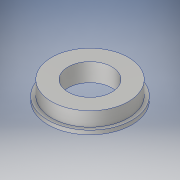
# Autodesk Inventor part: F6801_2019
Saved by Autodesk Inventor 2019.4 (Build 234330000, 330)
## iProperties
Created: 2020-02-07
Part Number: F6801_2019
Material: Aluminum 6061
Document SubType Name: Modeling
Designer: Paul Lefeuvre
Density: 2.7 g/cm^3
Appearance: Aluminum - Flat
Author: Paul Lefeuvre
Autodesk Inventor part; units mm, degrees
ref_plane "YZ Plane" through (0, 0, 0) normal (1, 0, 0) x (0, 1, 0)
ref_plane "XZ Plane" through (0, 0, 0) normal (0, 1, 0) x (-1, 0, 0)
ref_plane "XY Plane" through (0, 0, 0) normal (0, 0, 1) x (1, 0, 0)
sketch "Sketch1" plane through (0, 0, 0) normal (0, 0, 1) x (1, 0, 0)
  line L0 (6, 0) -> (11.5, 0)
  line L1 (11.5, 0) -> (11.5, 1.1)
  line L2 (6, 5) -> (10.5, 5)
  line L3 (10.5, 5) -> (10.5, 1.1)
  line L4 (10.5, 1.1) -> (11.5, 1.1)
  line L5 (0, 5) -> (0, 0)
  line L6 (6, 5) -> (6, 0)
  dimension "d0" = 11.5
  dimension "d1" = 1.1
  dimension "d2" = 10.5
  dimension "d3" = 3.9
  dimension "d4" = 6
  constraints: 14 end point, 5 perpendicular, 2 horizontal, 2 point on line
  measures "d0" distance of L5.end L0.end
  measures "d1" distance of L0.end L1.end
  measures "d2" distance of L5.start L2.end
  measures "d3" distance of L2.end L3.end
  measures "d4" distance between parallel lines of L5 L6
revolve "Revolution1" add sketch "Sketch1" angle 360 about axis through (0, 5, 0) along (0, -1, 0)
body "Solid1"
